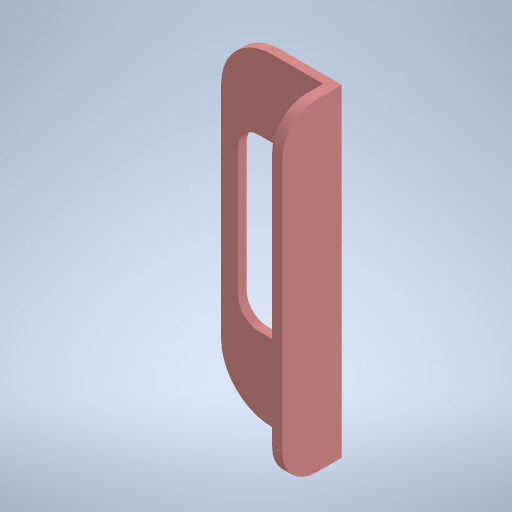
# Autodesk Inventor part: screen_back_support_right
Saved by Autodesk Inventor 2024 (Build 280153000, 153)
## iProperties
Created: 2024-02-15
Part Number: screen_back_support_right
Material: Generic
Document SubType Name: Modeling
Designer: fabiancastano
Density: 1 g/cm^3
Appearance: Default
Author: fabiancastano
Autodesk Inventor part; units mm, degrees
ref_plane "YZ Plane" through (0, 0, 0) normal (1, 0, 0) x (0, 1, 0)
ref_plane "XZ Plane" through (0, 0, 0) normal (0, 1, 0) x (-1, 0, 0)
ref_plane "XY Plane" through (0, 0, 0) normal (0, 0, 1) x (1, 0, 0)
sketch "Sketch1" plane through (0, 0, 0) normal (0, 0, 1) x (1, 0, 0)
  circle A0 centre (-3.0223, 127.0774) radius 1.5 projected
  circle A1 centre (-3.0236, 60.0769) radius 1.5 projected
  circle A2 centre (-3.0223, 127.0774) radius 1.5
  circle A3 centre (-3.0236, 60.0769) radius 1.5
  line L0 (3.5721, 158.6605) -> (3.572, -21.7605) projected
  line L1 (0.5721, 162.401) -> (0.572, -18.02)
  line L2 (0.572, 142.0774) -> (-14.428, 142.0774)
  line L3 (-29.428, 127.0774) -> (-29.428, 62.0774)
  line L4 (-14.428, 47.0774) -> (0.572, 47.0774)
  line L5 (0.572, 47.0774) -> (0.572, 142.0774)
  arc A4 (-14.428, 142.0774) -> (-29.428, 127.0774) centre (-14.428, 127.0774) ccw
  arc A5 (-29.428, 62.0774) -> (-14.428, 47.0774) centre (-14.428, 62.0774) ccw
  line L6 (-18.428, 119.5774) -> (-10.4279, 119.5774)
  line L7 (-4.428, 113.5774) -> (-4.428, 75.5774)
  line L8 (-10.428, 69.5774) -> (-18.428, 69.5774)
  line L9 (-24.428, 75.5774) -> (-24.428, 113.5774)
  arc A6 (-18.428, 119.5774) -> (-24.428, 113.5774) centre (-18.428, 113.5774) ccw
  arc A7 (-4.428, 113.5774) -> (-10.4279, 119.5774) centre (-10.4279, 113.5774) ccw
  arc A8 (-24.428, 75.5774) -> (-18.428, 69.5774) centre (-18.428, 75.5774) ccw
  arc A9 (-10.428, 69.5774) -> (-4.428, 75.5774) centre (-10.428, 75.5774) ccw
  line L10 (0.572, 142.0774) -> (3.572, 142.0774)
  line L11 (3.572, 142.0774) -> (3.572, 47.0774)
  line L12 (3.572, 47.0774) -> (0.572, 47.0774)
  line L13 (0.572, 47.0774) -> (0.572, 142.0774)
  point P0 (0, 0)
  point P1 (-29.428, 47.0774)
  point P2 (-29.428, 142.0774)
  point P3 (-24.428, 119.5774)
  point P4 (-4.428, 119.5774)
  point P5 (-24.428, 69.5774)
  point P6 (-24.428, 94.5774)
  point P7 (-29.428, 94.5774)
  point P8 (-14.428, 119.5774)
  point P9 (0.572, 47.0774)
  dimension "d0" = 3
  dimension "d1" = 30
  dimension "d2" = 95
  dimension "d3" = 15
  dimension "d4" = 15
  dimension "d7" = 50
  dimension "d8" = 20
  dimension "d9" = 6
  dimension "d10" = 95
  constraints: 26 end point, 12 point on circle, 12 point on line, 12 tangent, 8 centre point, 7 parallel, 6 equal radius, 3 horizontal, 3 midpoint, 3 perpendicular, 2 coincident, 1 horizontal alignment, 1 vertical alignment
  measures "d0" distance between parallel lines of L0 L1
  measures "d1" distance of L4.end point (-29.428, 47.077)
  measures "d2" distance of point (-29.428, 47.077) point (-29.428, 142.077)
  measures "d3" distance from line of L2 A0.centre
  measures "d4" radius of A4
  measures "d7" distance of point (-24.428, 69.577) point (-24.428, 119.577)
  measures "d8" distance of point (-24.428, 119.577) point (-4.428, 119.577)
  measures "d9" radius of A6
  measures "d10" distance of L10.end L11.end
extrude "Extrusion1" add sketch "Sketch1" along normal blind 2.5 contours L1 L4 A5 L3 A4 L2
sketch "Sketch2" plane through (0, 0, 2.5) normal (0, 0, 1) x (1, 0, 0)
  line L0 (0.572, 47.0774) -> (0.572, 142.0774) projected
  line L1 (0.572, 142.0774) -> (3.572, 142.0774)
  line L2 (3.572, 142.0774) -> (3.572, 47.0774)
  line L3 (3.572, 47.0774) -> (0.572, 47.0774)
  line L4 (0.572, 47.0774) -> (0.572, 142.0774)
  point P0 (0, 0)
  dimension "d13" = 3
  constraints: 8 end point, 2 parallel, 1 horizontal, 1 perpendicular
  measures "d13" distance of L2.end L3.end
extrude "Extrusion2" add sketch "Sketch2" along normal blind 15
fillet "Fillet1" radius 10 2 edges at (2.072, 47.0774, 17.5) (2.072, 142.0774, 17.5)
extrude "Extrusion3" add sketch "Sketch2" against normal blind 2.5
body "Solid1"
